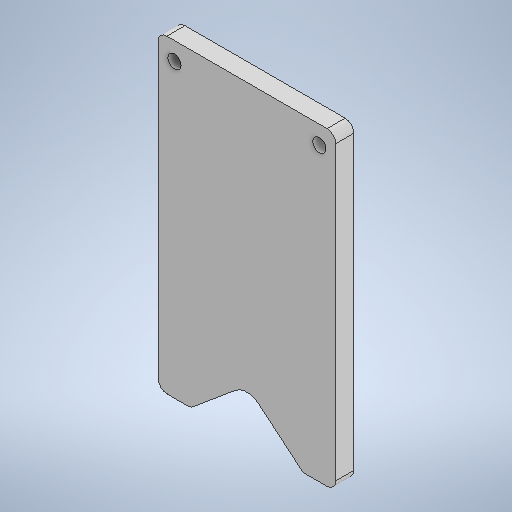
# Autodesk Inventor part: hinge align mech
Saved by Autodesk Inventor 2025.1 (Build 291241020, 241B)
## iProperties
Created: 2025-01-14
Part Number: hinge align mech
Material: Generic
Document SubType Name: Modeling
Designer: Hunter Mathis
Density: 1 g/cm^3
Appearance: Default
Author: Hunter Mathis
Autodesk Inventor part; units mm, degrees
ref_plane "YZ Plane" through (0, 0, 0) normal (1, 0, 0) x (0, 1, 0)
ref_plane "XZ Plane" through (0, 0, 0) normal (0, 1, 0) x (-1, 0, 0)
ref_plane "XY Plane" through (0, 0, 0) normal (0, 0, 1) x (1, 0, 0)
sketch "Sketch1" plane through (0, 0, 0) normal (0, 0, 1) x (1, 0, 0)
  line L0 (-24.765, 6.35) -> (24.765, 6.35)
  line L1 (24.765, 6.35) -> (24.765, -6.35)
  line L2 (24.765, -6.35) -> (-24.765, -6.35)
  line L3 (-24.765, -6.35) -> (-24.765, 6.35)
  line L4 (-24.765, 6.35) -> (24.765, -6.35) construction
  line L5 (24.765, 6.35) -> (-24.765, -6.35) construction
  point P0 (0, 0)
  dimension "d0" = 49.53
  dimension "d1" = 12.7
  constraints: 12 end point, 2 midpoint, 2 parallel, 1 horizontal, 1 perpendicular
  measures "d0" distance of L1.end L2.end
  measures "d1" distance of L0.end L1.end
extrude "Extrusion1" add sketch "Sketch1" along normal blind 3.175
sketch "Sketch4" plane through (24.765, -6.35, 0) normal (1, 0, 0) x (0, 0, -1)
  line L0 (-3.175, 0) -> (0, 0)
  line L1 (0, 0) -> (0, 12.7)
  line L2 (0, 12.7) -> (-3.175, 12.7)
  line L3 (-3.175, 12.7) -> (-3.175, 0)
  point P0 (0, 6.35)
  constraints: 8 end point, 2 parallel, 1 horizontal, 1 perpendicular
extrude "Extrusion4" add sketch "Sketch4" along normal blind 12.7
fillet "Fillet1" [suppressed]
sketch "Sketch5" plane through (0, 0, 0) normal (0, 0, -1) x (-1, 0, 0)
  arc A0 (25.4, 4.7625) -> (23.8125, 6.35) centre (23.8125, 4.7625) ccw projected
  line L0 (25.4, 4.7625) -> (25.4, 0)
  line L1 (25.4, 4.7625) -> (25.4, -4.7625) projected
  line L2 (25.4, 0) -> (19.05, 0)
  circle A1 centre (19.05, 0) radius 2.3241
  line L3 (23.8125, -6.35) -> (-36.5125, -6.35) construction
  circle A2 centre (6.35, 0) radius 2.3241
  circle A3 centre (-6.35, 0) radius 2.3241
  circle A4 centre (-19.05, 0) radius 2.3241
  circle A5 centre (-31.75, 0) radius 2.3241
  line L4 (23.8125, -6.35) -> (-36.5125, -6.35) projected
  line L5 (23.8125, -6.35) -> (-36.5125, -6.35) construction
  point P0 (0, 0)
  dimension "d33" = 6.35
  dimension "d34" = 4.6482
  dimension "d37" = 12.7
  constraints: 5 centre point, 4 end point, 1 coincident, 1 horizontal, 1 midpoint, 1 perpendicular, 8 other
  measures "d33" distance of L0.end L2.end
  measures "d34" diameter of A1
  measures "d37" distance of A1.centre A2.centre
extrude "Extrusion5" cut sketch "Sketch5" against normal blind 6.35 contours A1 | A5
sketch "Sketch6" plane through (-24.765, -6.35, 0) normal (0, -1, 0) x (1, 0, 0)
  line L0 (0, 0) -> (0, 3.175) projected
  line L1 (0, 0) -> (62.23, 0) projected
  line L2 (0, 3.175) -> (62.23, 3.175)
  line L3 (62.23, 3.175) -> (62.23, 0)
  line L4 (62.23, 0) -> (0, 0)
  line L5 (0, 0) -> (0, 3.175)
  point P0 (24.765, 0)
  constraints: 8 end point, 2 parallel, 1 horizontal, 1 perpendicular
extrude "Extrusion6" add sketch "Sketch6" along normal blind 41.91
fillet "Fillet2" [suppressed]
sketch "Sketch9" plane through (0, 0, 3.175) normal (0, 0, 1) x (1, 0, 0)
  line L0 (-25.4, -45.085) -> (-25.4, -32.385)
  line L1 (-25.4, -32.385) -> (38.1, -32.385)
  line L2 (37.465, 6.35) -> (37.465, -48.26) projected
  line L3 (38.1, -32.385) -> (38.1, -45.085)
  line L4 (-24.765, -48.26) -> (37.465, -48.26) projected
  line L5 (34.925, -48.26) -> (-22.225, -48.26)
  arc A0 (-25.4, -45.085) -> (-22.225, -48.26) centre (-22.225, -45.085) ccw
  arc A1 (34.925, -48.26) -> (38.1, -45.085) centre (34.925, -45.085) ccw
  line L6 (-24.765, 6.35) -> (-24.765, -48.26) projected
  line L7 (-25.4, -45.085) -> (-25.4, -48.26)
  line L8 (-22.225, -48.26) -> (-24.765, -48.26)
  line L9 (-25.4, -45.085) -> (-25.4, -48.26)
  line L10 (34.925, -48.26) -> (37.465, -48.26)
  line L11 (38.1, -48.26) -> (38.1, -45.085)
  point P0 (0, 0)
  point P1 (37.465, -32.385)
  point P2 (-24.765, -32.385)
  dimension "d54" = 12.7
  constraints: 18 end point, 4 point on circle, 4 tangent, 3 collinear, 3 perpendicular, 3 vertical, 2 centre point, 4 other
  measures "d54" distance of L0.start L0.end
extrude "Extrusion9" add sketch "Sketch9" along normal blind 3.175 contours L6 L1 L2 A1 L4 A0 | A0 L4 L6 | A1 L2 L4
fillet "Fillet3" [suppressed]
sketch "Sketch10" plane through (-24.765, -48.26, 0) normal (0, -1, 0) x (1, 0, 0)
  point P0 (24.765, 0)
sketch "Sketch11" plane through (-24.765, -48.26, 0) normal (0, -1, 0) x (1, 0, 0)
  line L0 (0, 0) -> (0, 6.35) projected
  line L1 (0, 6.35) -> (62.23, 6.35)
  line L2 (62.23, 6.35) -> (62.23, 0)
  line L3 (62.23, 0) -> (0, 0)
  line L4 (0, 0) -> (0, 6.35)
  point P0 (24.765, 0)
  constraints: 8 end point, 2 parallel, 1 horizontal, 1 perpendicular
extrude "Extrusion10" add sketch "Sketch11" along normal blind 53.975
sketch "Sketch12" plane through (0, 0, 6.35) normal (0, 0, 1) x (1, 0, 0)
  line L0 (-24.765, -102.235) -> (37.465, -102.235) projected
  line L1 (-24.765, -102.235) -> (37.465, -102.235)
  line L2 (37.465, -102.235) -> (6.35, -102.235)
  line L3 (6.35, -102.235) -> (21.9075, -102.235)
  line L4 (-24.765, -102.235) -> (6.35, -102.235)
  line L5 (6.35, -102.235) -> (-9.2075, -102.235)
  line L6 (-24.765, 6.35) -> (-24.765, -102.235) projected
  line L7 (-9.2075, -102.235) -> (-24.765, -102.235)
  line L8 (-24.765, -102.235) -> (-13.335, -102.235)
  line L9 (-13.335, -102.235) -> (2.2732, -89.165)
  line L10 (37.465, -102.235) -> (26.035, -102.235)
  line L11 (26.035, -102.235) -> (10.4268, -89.165)
  arc A0 (10.4268, -89.165) -> (2.2732, -89.165) centre (6.35, -94.0335) ccw
  point P0 (0, 0)
  point P1 (-13.335, -102.235)
  point P2 (26.035, -102.235)
  dimension "d73" = 11.43
  dimension "d74" = 11.43
  dimension "d75" = 6.35
  constraints: 20 end point, 3 midpoint, 2 collinear, 2 point on circle, 2 point on line, 2 tangent, 1 centre point, 1 horizontal
  measures "d73" distance of L0.start L8.end
  measures "d74" distance of L0.end L10.end
  measures "d75" radius of A0
extrude "Extrusion11" cut sketch "Sketch12" against normal through all
fillet "Fillet4" radius 3.175 2 edges at (-24.765, -102.235, 3.175) (37.465, -102.235, 3.175)
sketch "Sketch13" plane through (0, 0, 3.175) normal (0, 0, 1) x (1, 0, 0)
  line L0 (-24.765, 6.35) -> (37.465, 6.35) projected
  line L1 (-24.765, 6.35) -> (37.465, 6.35)
  line L2 (37.465, 6.35) -> (37.465, -32.385)
  line L3 (37.465, -32.385) -> (-24.765, -32.385)
  line L4 (-24.765, -32.385) -> (-24.765, 6.35)
  circle A0 centre (-19.05, 0) radius 2.3241 projected
  circle A1 centre (-19.05, 0) radius 2.3241
  circle A2 centre (31.75, 0) radius 2.3241 projected
  circle A3 centre (31.75, 0) radius 2.3241
  point P0 (0, 0)
  constraints: 8 end point, 2 centre point, 2 coincident, 2 parallel, 1 horizontal, 1 perpendicular
extrude "Extrusion12" add sketch "Sketch13" along normal up to surface (3.175 mm away) contours L0 L2 L3 L4 | A0 | A2
extrude "Extrusion13" cut sketch "Sketch13" along normal through all contours A0 | A2
fillet "Fillet7" radius 3.048 2 edges at (37.465, 6.35, 3.175) (-24.765, 6.35, 3.175)
fillet "Fillet8" radius 3.048 2 edges at (26.035, -102.235, 3.175) (-13.335, -102.235, 3.175)
body "Solid1"
